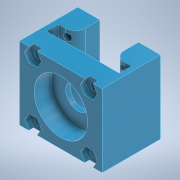
# Autodesk Inventor part: Tensor
Saved by Autodesk Inventor 2021 (Build 250183000, 183)
## iProperties
Created: 2022-10-27
Part Number: Tensor
Material: Generic
Document SubType Name: Modeling
Designer: USUARIO
Density: 1 g/cm^3
Appearance: Sky Blue Dark
Author: USUARIO
Autodesk Inventor part; units mm, degrees
ref_plane "YZ Plane" through (0, 0, 0) normal (1, 0, 0) x (0, 1, 0)
ref_plane "XZ Plane" through (0, 0, 0) normal (0, 1, 0) x (-1, 0, 0)
ref_plane "XY Plane" through (0, 0, 0) normal (0, 0, 1) x (1, 0, 0)
sketch "Sketch1" plane through (0, 0, 0) normal (0, 1, 0) x (-1, 0, 0)
  line L0 (0, -37.4557) -> (0, 23.9689) construction
  line L1 (8, -2) -> (8, -12)
  line L2 (8, -12) -> (17, -12)
  line L3 (17, -12) -> (17, 12)
  line L4 (17, 12) -> (0, 12)
  line L5 (8, -2) -> (15, -2)
  line L6 (15, -2) -> (15, 3)
  line L7 (15, 3) -> (0, 3)
  line L8 (0, -49.7407) -> (0, 36.2538) projected
  line L9 (-8, -2) -> (-8, -12)
  line L10 (-8, -12) -> (-17, -12)
  line L11 (-17, -12) -> (-17, 12)
  line L12 (-17, 12) -> (0, 12)
  line L13 (-8, -2) -> (-15, -2)
  line L14 (-15, -2) -> (-15, 3)
  line L15 (-15, 3) -> (0, 3)
  line L16 (23.8, 0) -> (-23.8, 0) projected
  point P0 (17, 0)
  point P1 (-17, 0)
  dimension "d12" = 15
  dimension "d13" = 5
  dimension "d14" = 7
  dimension "d15" = 10
  dimension "d16" = 9
  dimension "d18" = 9
  dimension "d19" = 17
  constraints: 30 end point, 7 symmetric about line, 3 parallel, 2 perpendicular, 2 point on line, 2 vertical, 1 collinear, 1 horizontal, 1 midpoint
  measures "d12" distance of L6.end L7.end
  measures "d13" distance of L5.end L6.end
  measures "d14" distance of L1.start L5.end
  measures "d15" distance of L1.start L1.end
  measures "d16" distance of L1.end L2.end
  measures "d18" distance between parallel lines of L4 L7
  measures "d19" distance of L3.end L4.end
extrude "Extrusion1" add sketch "Sketch1" along normal blind 30 contours L5 L6 L16 L3 L2 L1 | L6 L7 L8 L4 L3 L16 | L15 L14 L16 L11 L12 L8 | L14 L13 L9 L10 L11 L16
fillet "Fillet1" radius 4 2 edges at (-8, 15, -2) (8, 15, -2)
sketch "Sketch2" plane through (-17, 0, 12) normal (0, 0, 1) x (1, 0, 0)
  line L0 (0, 0) -> (34, 0) projected
  line L1 (34, 0) -> (34, 30) projected
  line L2 (0, 30) -> (34, 30) projected
  line L3 (0, 0) -> (0, 30) projected
  line L4 (34, 0) -> (34, 30) projected
  line L5 (34, 15) -> (0, 15) construction
  line L6 (0, 0) -> (0, 30) projected
  circle A0 centre (17, 15) radius 11
  circle A1 centre (17, 15) radius 5
  line L7 (0, 0) -> (34, 0) projected
  line L8 (5, 30) -> (5, 0) projected
  line L9 (2, 30) -> (5, 30) projected
  line L10 (2, 0) -> (2, 30) projected
  line L11 (2, 0) -> (5, 0) projected
  line L12 (29, 0) -> (29, 30) projected
  line L13 (29, 0) -> (32, 0) projected
  line L14 (32, 0) -> (32, 30) projected
  line L15 (29, 30) -> (32, 30) projected
  circle A2 centre (28.5, 27) radius 1.5
  line L16 (17, 15) -> (17, 38.5815) construction
  circle A3 centre (5.5, 27) radius 1.5
  circle A4 centre (28.5, 3) radius 1.5
  circle A5 centre (5.5, 3) radius 1.5
  point P0 (17, 0)
  dimension "d23" = 22
  dimension "d24" = 10
  dimension "d25" = 3
  dimension "d26" = 11.5
  dimension "d27" = 12
  constraints: 6 centre point, 4 end point, 3 midpoint, 3 symmetric about line, 1 coincident, 1 vertical, 3 other
  measures "d23" diameter of A0
  measures "d24" diameter of A1
  measures "d25" diameter of A2
  measures "d26" horizontal distance of A0.centre A2.centre
  measures "d27" vertical distance of A2.centre A0.centre
extrude "Extrusion2" cut sketch "Sketch2" against normal blind 7 contours A0
extrude "Extrusion3" cut sketch "Sketch2" against normal through all contours A5 L8 | L8 A5 | A4 L12 | L12 A4 | A3 L8 | L8 A3 | A2 L12 | L12 A2 | A1
sketch "Sketch3" plane through (-17, 0, 12) normal (0, 0, 1) x (1, 0, 0)
  circle A0 centre (28.5, 27) radius 1.5 projected
  line L0 (25.0359, 27) -> (26.7679, 30)
  line L1 (26.7679, 30) -> (30.2321, 30)
  line L2 (30.2321, 30) -> (31.9641, 27)
  line L3 (31.9641, 27) -> (30.2321, 24)
  line L4 (30.2321, 24) -> (26.7679, 24)
  line L5 (26.7679, 24) -> (25.0359, 27)
  circle A1 centre (17, 15) radius 5 projected
  line L6 (17, 15) -> (17, 32.2239) construction
  line L7 (17, 15) -> (37.5961, 15) construction
  line L8 (2.0359, 27) -> (3.7679, 30)
  line L9 (3.7679, 30) -> (7.2321, 30)
  line L10 (7.2321, 30) -> (8.9641, 27)
  line L11 (8.9641, 27) -> (7.2321, 24)
  line L12 (7.2321, 24) -> (3.7679, 24)
  line L13 (3.7679, 24) -> (2.0359, 27)
  line L14 (25.0359, 3) -> (26.7679, 6)
  line L15 (26.7679, 6) -> (30.2321, 6)
  line L16 (30.2321, 6) -> (31.9641, 3)
  line L17 (31.9641, 3) -> (30.2321, 0)
  line L18 (30.2321, 0) -> (26.7679, 0)
  line L19 (26.7679, 0) -> (25.0359, 3)
  line L20 (2.0359, 3) -> (3.7679, 6)
  line L21 (3.7679, 6) -> (7.2321, 6)
  line L22 (7.2321, 6) -> (8.9641, 3)
  line L23 (8.9641, 3) -> (7.2321, 0)
  line L24 (7.2321, 0) -> (3.7679, 0)
  line L25 (3.7679, 0) -> (2.0359, 3)
  point P0 (17, 0)
  dimension "d32" = 6
  dimension "d35" = 23
  dimension "d38" = 24
  constraints: 52 end point, 3 horizontal, 2 vertical, 1 coincident, 49 other
  measures "d32" distance between parallel lines of L4 L1
  measures "d35" distance of L0.start L8.start
  measures "d38" distance of L0.start L14.start
extrude "Extrusion4" cut sketch "Sketch3" against normal blind 2 contours L0 L1 L2 L3 L4 L5 | L8 L9 L10 L11 L12 L13 | L14 L15 L16 L17 L18 L19 | L20 L21 L22 L23 L24 L25
body "Solid1"
